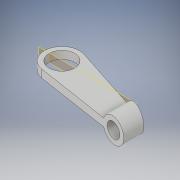
# Autodesk Inventor part: motor test flapper nema23
Saved by Autodesk Inventor 2018.2 (Build 222227000, 227)
## iProperties
Created: 2018-03-04
Part Number: motor test flapper nema23
Material: Generic
Document SubType Name: Modeling
Designer: torba
Density: 1 g/cm^3
Appearance: Default
Author: torba
Autodesk Inventor part; units mm, degrees
ref_plane "YZ Plane" through (0, 0, 0) normal (1, 0, 0) x (0, 1, 0)
ref_plane "XZ Plane" through (0, 0, 0) normal (0, 1, 0) x (-1, 0, 0)
sketch "Sketch11" plane through (0, 0, 0) normal (0, 1, 0) x (-1, 0, 0)
  circle A0 centre (-0.7928, 0.0539) radius 8.2
  line L0 (-60.6518, 3.7281) -> (-51.4268, 3.7281)
  circle A1 centre (-0.7928, 0.0539) radius 11.2
  line L1 (-51.4268, 3.7281) -> (-48.4268, 3.7281)
  line L2 (-60.6518, 3.7281) -> (-63.6518, 3.7281)
  line L3 (-48.4268, 3.7281) -> (-4.248, -10.5999)
  line L4 (-48.4268, 3.7281) -> (-48.4268, 18.7281)
  line L5 (-48.4268, 18.7281) -> (0.9133, 11.1231)
  point P0 (0, 0)
  point P1 (-55.4678, 32.9951)
  point P2 (-56.0393, 3.7281)
  dimension "d63" = 16.4
  dimension "d64" = 22.4
  dimension "d65" = 9.225
  dimension "d66" = 3
  dimension "d67" = 3
  dimension "d68" = 15
  dimension "d76" = 48.4268
  constraints: 12 end point, 2 centre point, 2 horizontal, 2 point on circle, 2 tangent, 1 coincident, 1 midpoint, 1 vertical
  measures "d63" diameter of A0
  measures "d64" diameter of A1
  measures "d65" distance of L0.start L0.end
  measures "d66" distance of L0.end L1.end
  measures "d67" distance of L0.start L2.end
  measures "d68" distance of L1.end L4.end
  measures "d76" distance from line of point (0, 0) L4
extrude "Extrusion9" add sketch "Sketch11" along normal blind 5
ref_plane "Work Plane2" through (0, 0, 0) normal (0, 0, 1) x (1, 0, 0)
sketch "Sketch12" plane through (0, 0, 0) normal (0, 0, 1) x (1, 0, 0)
  line L0 (48.4268, 0) -> (48.4268, 5) projected
  line L1 (48.4268, 0) -> (4.248, 0) projected
  line L2 (48.4268, 0) -> (4.248, 0) projected
  line L3 (4.248, 0) -> (4.248, 5) projected
  line L4 (48.4268, 5) -> (4.248, 5) projected
  line L5 (48.4268, 0) -> (48.4268, 5) projected
  line L6 (48.4268, 0) -> (48.4268, 5) projected
  line L7 (48.4268, 2.5) -> (53.1898, 2.5)
  circle A0 centre (53.1898, 2.5) radius 4.763
  circle A1 centre (53.1898, 2.5) radius 7.763
  point P0 (0, 0)
  dimension "d72" = 4.763
  dimension "d73" = 15.526
  constraints: 2 coincident, 2 end point, 1 centre point, 1 horizontal, 1 horizontal alignment, 1 midpoint, 2 other
  measures "d72" distance of L7.start L7.end
  measures "d73" diameter of A1
extrude "Extrusion10" add sketch "Sketch12" along normal up to surface contours L1 A1 L4 L0 | L0 L4 A1 L1 starts on plane at (48.4268, 0, 3.7281) facing (0.308499, 0, -0.9512247) surface through (-0.9133, 0, 11.1231) normal (-0.1523344, 0, 0.988329)
body "Solid3"
